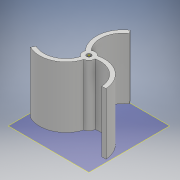
# Autodesk Inventor part: pump_impeller
Saved by Autodesk Inventor 2017 (Build 210142000, 142)
## iProperties
Created: 2016-12-23
Part Number: pump_impeller
Material: Generic
Document SubType Name: Modeling
Designer: Ali
Density: 1 g/cm^3
Appearance: Default
Author: Ali
Autodesk Inventor part; units mm, degrees
ref_plane "YZ Plane" through (0, 0, 0) normal (1, 0, 0) x (0, 1, 0)
ref_plane "XZ Plane" through (0, 0, 0) normal (0, 1, 0) x (-1, 0, 0)
ref_plane "XY Plane" through (0, 0, 0) normal (0, 0, 1) x (1, 0, 0)
ref_plane "Work Plane1" through (8.8633, 1.5628, -1) normal (0, 0, -1) x (-1, 0, 0)
sketch "Sketch1" plane through (8.8633, 1.5628, -1) normal (0, 0, -1) x (-1, 0, 0)
  circle A0 centre (8.8633, -1.5628) radius 1.5 projected
  circle A1 centre (8.8633, -1.5628) radius 0.55 projected
  point P0 (8.8633, -1.5628)
extrude "Extrusion1" add sketch "Sketch1" against normal blind 15
sketch "Sketch2" plane through (0, 0, 14) normal (0, 0, 1) x (1, 0, 0)
  circle A0 centre (0, 0) radius 1.5 projected
  line L0 (0.2764, 9.5833) -> (-0.2764, 10.4166)
  line L1 (8.1612, -5.0311) -> (9.1593, -4.969) projected
  line L2 (-8.4376, -4.5523) -> (-8.8829, -5.4477) projected
  arc A1 (8.1612, -5.0311) -> (1.5, 0.0014) centre (2.6718, -5.3723) ccw
  arc A2 (-8.4376, -4.5523) -> (-0.7487, -1.2998) centre (-5.9884, 0.3723) ccw
  arc A3 (-8.8829, -5.4477) -> (0.242, -1.4803) centre (-5.9884, 0.3723) ccw
  line L3 (-8.8829, -5.4477) -> (-8.4376, -4.5523)
  line L4 (8.1612, -5.0311) -> (9.1593, -4.969)
  circle A4 centre (3.3166, 4.9999) radius 5.4999 projected
  circle A5 centre (3.3165, 4.9999) radius 6.4999 projected
  circle A6 centre (2.6718, -5.3723) radius 5.5 projected
  circle A7 centre (2.6718, -5.3725) radius 6.5001 projected
  circle A8 centre (-5.9884, 0.3723) radius 6.5 projected
  circle A9 centre (-5.9884, 0.3721) radius 5.4999 projected
  arc A10 (-0.2764, 10.4166) -> (-1.403, 0.5306) centre (3.3167, 5) ccw
  arc A11 (0.2764, 9.5833) -> (-0.7512, 1.2983) centre (3.3167, 5) ccw
  arc A12 (9.1593, -4.969) -> (1.161, 0.9497) centre (2.6718, -5.3723) ccw
  point P0 (0, 0)
  point P1 (-2.459, 2.3282)
  constraints: 18 point on circle, 6 centre point, 6 end point, 1 other
extrude "Extrusion2" add sketch "Sketch2" against normal blind 15 contours A0 A7 A4 A1 | A4 A7 A5 A1 | A5 A7 L1 A1 | A8 A5 L0 A4 | A4 A9 A5 A8 | A3 A6 A2 A0 | A0 A5 A9 A4 | A3 A7 A2 A6 | L2 A2 A7 A3
sketch "Sketch4" plane through (8.8633, 1.5628, 14) normal (0, 0, 1) x (1, 0, 0)
  point P0 (-8.8633, -1.5628)
body "Solid1"
